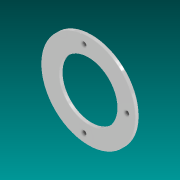
# Autodesk Inventor part: AxiaalLagerBevestiging
Saved by Autodesk Inventor 2020.2 (Build 242310000, 310)
## iProperties
Created: 2020-05-15
Part Number: AxiaalLagerBevestiging
Material: Aluminum 6061
Document SubType Name: Modeling
Designer: Svend
Density: 2.7 g/cm^3
Appearance: Aluminum - Polished
Author: Svend
Autodesk Inventor part; units mm, degrees
ref_plane "YZ Plane" through (0, 0, 0) normal (1, 0, 0) x (0, 1, 0)
ref_plane "XZ Plane" through (0, 0, 0) normal (0, 1, 0) x (-1, 0, 0)
ref_plane "XY Plane" through (0, 0, 0) normal (0, 0, 1) x (1, 0, 0)
sketch "Sketch1" plane through (0, 0, 0) normal (0, 0, 1) x (1, 0, 0)
  circle A0 centre (0, 0) radius 56.437
  circle A1 centre (0, 0) radius 35
  circle A2 centre (46.437, 0) radius 2.5
  circle A3 centre (0, 0) radius 11.5
  circle A4 centre (-5.0711, 46.1809) radius 2.5
  circle A5 centre (-5.0711, -46.1809) radius 2.5
  point P0 (46.4372, 0)
  dimension "d0" = 112.874
  dimension "d1" = 70
  dimension "d2" = 5
  dimension "d3" = 46.437
  dimension "d4" = 23
  dimension "d5" = 46.1809
  dimension "d6" = 46.4372
  dimension "d7" = 46.1809
  dimension "d8" = 5.0711
  dimension "d9" = 5.0711
  constraints: 6 centre point, 5 coincident, 2 equal radius, 2 horizontal alignment
  measures "d0" diameter of A0
  measures "d1" diameter of A1
  measures "d2" diameter of A2
  measures "d3" distance of point (0, 0) A2.centre
  measures "d4" diameter of A3
  measures "d5" vertical distance of point (-5.071, 46.181) A3.centre
  measures "d6" distance of point (46.437, 0) A3.centre
  measures "d7" vertical distance of point (-5.071, -46.181) A3.centre
  measures "d8" horizontal distance of point (-5.071, -46.181) A3.centre
  measures "d9" horizontal distance of point (-5.071, 46.181) A3.centre
extrude "Extrusion1" add sketch "Sketch1" along normal mid plane 4 contours A0
chamfer "Chamfer1" distance 0.2 angle 45 10 edges at (-56.437, 0, 2) (43.937, 0, 2) (-7.5711, -46.1809, 2) (-7.5711, 46.1809, 2) (-35, 0, 2) (-35, 0, -2) (-7.5711, 46.1809, -2) (-7.5711, -46.1809, -2) (43.937, 0, -2) (-56.437, 0, -2)
body "Solid1"
